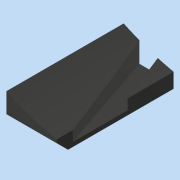
# Autodesk Inventor part: WireGuideToSail2
Saved by Autodesk Inventor 2017 (Build 210142000, 142)
## iProperties
Created: 2018-03-28
Part Number: WireGuideToSail2
Material: ABS Plastic
Document SubType Name: Modeling
Designer: Derek Wider
Density: 1.06 g/cm^3
Appearance: Smooth - Black
Author: Derek Wider
Autodesk Inventor part; units mm, degrees
ref_plane "YZ Plane" through (0, 0, 0) normal (1, 0, 0) x (0, 1, 0)
ref_plane "XZ Plane" through (0, 0, 0) normal (0, 1, 0) x (-1, 0, 0)
ref_plane "XY Plane" through (0, 0, 0) normal (0, 0, 1) x (1, 0, 0)
sketch "Sketch1" plane through (0, 0, 0) normal (0, 0, 1) x (1, 0, 0)
  line L0 (0, 6.831) -> (0, 0)
  line L1 (0, 0) -> (10.795, 0)
  line L2 (10.795, 0) -> (10.795, 3.175)
  arc A0 (0, 6.831) -> (10.795, 3.175) centre (21.59, 52.8148) ccw
  line L3 (10.795, 3.175) -> (21.59, 3.175) construction
  line L4 (21.59, 3.175) -> (21.59, 2.0148) construction
  arc A1 (10.795, 3.175) -> (21.59, 2.0148) centre (21.59, 52.8148) ccw construction
  dimension "d0" = 50.8
  dimension "d4" = 10.795
  dimension "d12" = 3.175
  dimension "d13" = 10.795
  constraints: 10 end point, 4 point on circle, 3 perpendicular, 2 centre point, 1 coincident, 1 concentric, 1 horizontal, 1 line through centre, 1 point on line, 1 vertical
  measures "d0" radius of A0
  measures "d4" distance of L0.end L1.end
  measures "d12" distance of L1.end L2.end
  measures "d13" distance of L2.end L3.end
extrude "Extrusion1" add sketch "Sketch1" along normal blind 25.4
ref_plane "Work Plane1" through (0, 3.175, 0) normal (0, -1, 0) x (1, 0, 0)
sketch "Sketch2" plane through (0, 3.175, 0) normal (0, -1, 0) x (1, 0, 0)
  line L0 (0, 0) -> (0, 25.4) projected
  line L1 (10.795, 15.875) -> (5.3975, 0)
  line L2 (10.795, 0) -> (0, 0) projected
  line L3 (0, 25.4) -> (10.795, 25.4) projected
  line L4 (10.795, 0) -> (10.795, 25.4) projected
  line L5 (10.795, 0) -> (10.795, 25.4) projected
  dimension "d14" = 9.525
  constraints: 2 end point, 2 point on line, 1 midpoint
  measures "d14" distance of L1.start L3.end
ref_plane "Work Plane2" through (10.795, 3.175, 15.875) normal (-0.3219027, 0, -0.9467727) x (0, 1, 0)
sketch "Sketch3" plane through (10.795, 3.175, 15.875) normal (-0.3219027, 0, -0.9467727) x (0, 1, 0)
  line L0 (2.2225, -1.905) -> (-2.2225, -1.905)
  line L1 (-2.2225, -1.905) -> (-2.2225, 1.905)
  line L2 (-2.2225, 1.905) -> (2.2225, 1.905)
  line L3 (2.2225, 1.905) -> (2.2225, -1.905)
  point P0 (-3.175, -5.1102)
  point P1 (0, 0)
  point P2 (2.2225, 0)
  point P3 (0, 1.905)
  dimension "d7" = 4.445
  dimension "d10" = 3.81
  constraints: 8 end point, 2 midpoint, 2 parallel, 1 horizontal, 1 horizontal alignment, 1 perpendicular, 1 vertical alignment
  measures "d7" distance of L0.start L0.end
  measures "d10" distance of L0.end L1.end
extrude "Extrusion2" cut sketch "Sketch3" along normal through all both and the other way through all
chamfer "Chamfer1" distance 2.54 angle 45 1 edges at (0, 0, 12.7)
chamfer "Chamfer2" distance 2.54 angle 45 1 edges at (6.6675, 0, 25.4)
body "Solid1"
